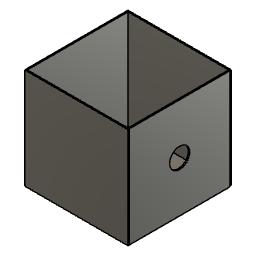
Rotating Flag Toy (Autodesk Fusion 360 archive; units mm, degrees)
design "gear1"
Autodesk Fusion 360 part; units mm, degrees
sketch "Sketch1" plane through (0, 0, 0) normal (0, 1, 0) x (1, 0, 0)
  line L0 (0, 0) -> (100, 0)
  line L1 (100, 0) -> (100, -100)
  line L2 (100, -100) -> (0, -100)
  line L3 (0, -100) -> (0, 0)
  constraint horizontal L0
  constraint vertical L1
  constraint horizontal L2
  constraint vertical L3
  constraint coincident L0.start L3.end
sketch "Sketch2" plane through (0, 0, 0) normal (0, 1, 0) x (1, 0, 0)
  line L0 (0, 0) -> (100, 0)
  line L1 (100, 0) -> (100, -100)
  line L2 (100, -100) -> (0, -100)
  line L3 (0, -100) -> (0, 0)
  constraint horizontal L0
  constraint vertical L1
  constraint horizontal L2
  constraint vertical L3
  constraint coincident L0.start L3.end
sketch "Sketch3" plane through (0, 0, 0) normal (0, 1, 0) x (1, 0, 0)
  line L0 (0, 0) -> (150, 0)
  line L1 (150, 0) -> (150, -150)
  line L2 (150, -150) -> (0, -150)
  line L3 (0, -150) -> (0, 0)
  dimension "d5" = 150
  dimension "d6" = 150
  constraint horizontal L0
  constraint vertical L1
  constraint horizontal L2
  constraint vertical L3
  constraint coincident L0.start L3.end
  measures "d5" distance of L0.start L0.end
  measures "d6" distance of L0.start L2.end
extrude "Extrude3" add sketch "Sketch3" along normal blind 2 makes body 1
sketch "Sketch4" plane through (150, 0, 0) normal (1, 0, 0) x (0, 0, -1)
  line L0 (-150, 0) -> (0, 0)
  line L1 (0, 0) -> (0, 2)
  line L2 (0, 2) -> (-150, 2)
  line L3 (-150, 2) -> (-150, 0)
  line L4 (0, 0) -> (-150, 0)
  line L5 (-150, 0) -> (-150, 150)
  line L6 (-150, 150) -> (0, 150)
  line L7 (0, 150) -> (0, 0)
  dimension "d9" = 150
  dimension "d10" = 150
  constraint horizontal L4
  constraint vertical L5
  constraint horizontal L6
  constraint vertical L7
  constraint coincident L0.end L1.start
  measures "d9" distance of L0.end L0.start
  measures "d10" distance of L0.end L6.end
extrude "Extrude4" add sketch "Sketch4" along normal blind 2 separate body contours L2 L5 L6 L7 makes body 2
move_face "OffsetFaces1" offset 2 1 faces at (151.3333, 2, 50) on bodies 2
sketch "Sketch5" plane through (0, 0, 0) normal (1, 0, 0) x (0, 0, -1)
  line L0 (0, 0) -> (-150, 0)
  line L1 (-150, 0) -> (-150, 150)
  line L2 (-150, 150) -> (0, 150)
  line L3 (0, 150) -> (0, 0)
  dimension "d14" = 150
  dimension "d15" = 150
  constraint horizontal L0
  constraint vertical L1
  constraint horizontal L2
  constraint vertical L3
  constraint coincident L0.start L3.end
  measures "d14" distance of L0.start L0.end
  measures "d15" distance of L0.start L2.end
extrude "Extrude5" add sketch "Sketch5" against normal blind 2 bodies 1
sketch "Sketch6" plane through (0, 0, 0) normal (0, 0, 1) x (1, 0, 0)
  line L0 (151.9625, 0.9965) -> (-1.993, 0.9965)
  line L1 (-1.993, 0.9965) -> (-1.993, 149.9695)
  line L2 (-1.993, 149.9695) -> (151.9625, 149.9695)
  line L3 (151.9625, 149.9695) -> (151.9625, 0.9965)
  constraint horizontal L0
  constraint vertical L1
  constraint horizontal L2
  constraint vertical L3
extrude "Extrude6" add sketch "Sketch6" against normal blind 2 bodies 1 2
ref_plane "WorkPlane1" through (0, 0, 150) normal (0, 0, 1) x (1, 0, 0)
sketch "Sketch7" plane through (0, 0, 150) normal (0, 0, 1) x (1, 0, 0)
  line L0 (0, 0) -> (151.9611, 0)
  line L1 (151.9611, 0) -> (151.9611, 149.9617)
  line L2 (151.9611, 149.9617) -> (0, 149.9617)
  line L3 (0, 149.9617) -> (0, 0)
  constraint horizontal L0
  constraint vertical L1
  constraint horizontal L2
  constraint vertical L3
  constraint coincident L0.start L3.end
extrude "Extrude7" add sketch "Sketch7" along normal blind 2 separate body makes body 3
move_face "OffsetFaces2" offset 2 1 faces at (0, 99.9744, 150.6667) on bodies 3
hole "Hole1" at (152, 75, 75) direction (-1, 0, 0) diameter 30 depth 50 tip angle 118 bodies 1

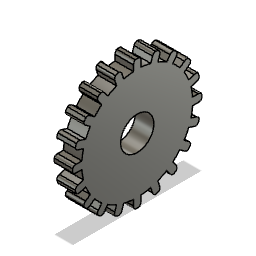
design "gear6"
Autodesk Fusion 360 part; units mm, degrees
sketch "Sketch1" plane through (0, 0, 0) normal (1, 0, 0) x (0, 0, -1)
  circle A0 centre (0, 0) radius 30
  dimension "d1" = 60
  constraint coincident A0.centre origin
  measures "d1" diameter of A0
extrude "Extrude1" add sketch "Sketch1" along normal blind 10
sketch "Sketch2" plane through (10, 0, 0) normal (1, 0, 0) x (0, 0, -1)
  circle A0 centre (0, 0) radius 30
  line L0 (-2.0249, 29.9316) -> (-2.0249, 33.0252)
  arc A1 (-1.0479, 34.9796) -> (-2.0249, 33.0252) centre (0.4183, 33.0252) ccw
  line L1 (-1.0479, 34.9796) -> (0.9463, 34.9796)
  arc A2 (2.0432, 33.0065) -> (0.9463, 34.9796) centre (0.0824, 33.2079) ccw
  line L2 (2.0432, 33.0065) -> (2.0432, 29.9303)
  constraint coincident A0 L0.start
  constraint vertical L0
  constraint tangent L0 A1
  constraint horizontal L1
  constraint coincident A0 L2.end
  constraint vertical L2
extrude "Extrude2" add sketch "Sketch2" against normal blind 10 contours A0 L0 A1 L1 A2 L2
pattern_circular "C-Pattern1" count 20 over 360 about axis through (0, 0, 0) along (1, 0, 0) of "Extrude2"
hole "Hole1" at (10, 0, 0) direction (-1, 0, 0) diameter 18 depth 18 tip angle 118

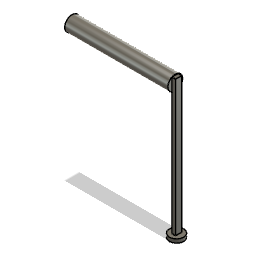
design "gear4"
Autodesk Fusion 360 part; units mm, degrees
sketch "Sketch1" plane through (0, 0, 0) normal (1, 0, 0) x (0, 0, -1)
  circle A0 centre (-15.9104, 20.2251) radius 10
  dimension "d1" = 20
  measures "d1" diameter of A0
extrude "Extrude1" add sketch "Sketch1" along normal blind 140
sketch "Sketch2" plane through (140, 0, 0) normal (1, 0, 0) x (0, 0, -1)
  circle A0 centre (-15.9104, 20.2251) radius 10
  line L0 (-20.4358, 29.1425) -> (-12.1034, 29.1425)
  line L1 (-12.1034, 29.1425) -> (-12.1034, -29.774)
  line L2 (-12.1034, -29.774) -> (-20.4358, -29.774)
  line L3 (-20.4358, -29.774) -> (-20.4358, 29.1425)
  constraint horizontal L0
  constraint vertical L1
  constraint horizontal L2
  constraint vertical L3
  constraint coincident A0 L0.start
extrude "Extrude2" add sketch "Sketch2" along normal blind 5 contours A0 L0 L1 L3 | A0 L1 L2 L3
extrude "Extrude3" add 1 faces at (141.6667, -29.774, 14.8809) along direction (0, -1, 0) blind 125
sketch "Sketch3" plane through (0, -154.774, 0) normal (0, -1, 0) x (1, 0, 0)
  line L0 (140, 20.4358) -> (140, 12.1034)
  line L1 (140, 12.1034) -> (145, 12.1034)
  line L2 (145, 12.1034) -> (145, 20.4358)
  line L3 (145, 20.4358) -> (140, 20.4358)
  circle A0 centre (142.5, 16.588) radius 9.71
extrude "Extrude4" add sketch "Sketch3" along normal blind 5 contours L0 L1 L2 L3 | A0

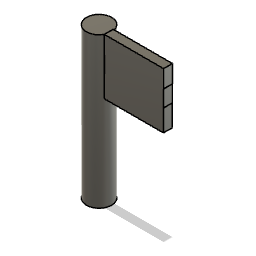
design "flag"
Autodesk Fusion 360 part; units mm, degrees
sketch "Sketch1" plane through (0, 0, 0) normal (0, 1, 0) x (1, 0, 0)
  circle A0 centre (0, 0) radius 4.263
  dimension "d1" = 8.526
  constraint coincident A0.centre origin
  measures "d1" diameter of A0
extrude "Extrude1" add sketch "Sketch1" along normal blind 51 makes body 1
sketch "Sketch2" plane through (0, 0, 0) normal (0, 0, 1) x (1, 0, 0)
  line L0 (4.2735, 51.0087) -> (19.9199, 51.0087)
  line L1 (19.9199, 51.0087) -> (19.9199, 45.0265)
  line L2 (19.9199, 45.0265) -> (4.2735, 45.0265)
  line L3 (4.2735, 45.0265) -> (4.2735, 51.0087)
  line L4 (4.2735, 45.0265) -> (19.9199, 45.0265)
  line L5 (19.9199, 45.0265) -> (19.9199, 39.038)
  line L6 (19.9199, 39.038) -> (4.2735, 39.038)
  line L7 (4.2735, 39.038) -> (4.2735, 45.0265)
  line L8 (4.2735, 39.038) -> (19.9199, 39.038)
  line L9 (19.9199, 39.038) -> (19.9199, 32.9058)
  line L10 (19.9199, 32.9058) -> (4.2735, 32.9058)
  line L11 (4.2735, 32.9058) -> (4.2735, 39.038)
  constraint horizontal L0
  constraint vertical L1
  constraint horizontal L2
  constraint vertical L3
  constraint horizontal L4
  constraint vertical L5
  constraint horizontal L6
  constraint vertical L7
  constraint horizontal L8
  constraint vertical L9
  constraint horizontal L10
  constraint vertical L11
extrude "Extrude2" add sketch "Sketch2" along normal blind 2 separate body contours L0 L1 L2 L3 L4 makes body 2
extrude "Extrude3" add 1 faces at (14.7044, 49.0146, 0) along direction (0, 0, -1) blind 1 on bodies 2 bodies 2
move_face "OffsetFaces1" offset 16 1 faces at (19.9199, 49.0146, 0) on bodies 2
move_face "OffsetFaces2" offset -12 1 faces at (35.9199, 49.0146, 0) on bodies 2
sketch "Sketch3" plane through (0, 0, 0) normal (0, 0, 1) x (1, 0, 0)
  line L0 (4.2852, 45.0296) -> (23.8847, 45.0296)
  line L1 (23.8847, 45.0296) -> (23.8847, 39.4097)
  line L2 (23.8847, 39.4097) -> (4.2852, 39.4097)
  line L3 (4.2852, 39.4097) -> (4.2852, 45.0296)
  constraint horizontal L0
  constraint vertical L1
  constraint horizontal L2
  constraint vertical L3
extrude "Extrude4" add sketch "Sketch3" along normal blind 2 bodies 2
move_face "OffsetFaces3" offset 1 1 faces at (10.8183, 43.1542, 0) on bodies 2
extrude "Extrude5" add 1 faces at (4.2852, 43.1542, 1) along direction (-1, 0, 0) blind 0.5 on bodies 2 bodies 2 1
extrude "Extrude6" add 1 faces at (4.2735, 47.0206, 0) along direction (-1, 0, 0) blind 0.5 on bodies 2 bodies 2
sketch "Sketch4" plane through (0, 0, 0) normal (0, 0, 1) x (1, 0, 0)
  line L0 (3.7832, 39.4209) -> (23.8708, 39.4209)
  line L1 (23.8708, 39.4209) -> (23.8708, 32.0868)
  line L2 (23.8708, 32.0868) -> (3.7832, 32.0868)
  line L3 (3.7832, 32.0868) -> (3.7832, 39.4209)
  constraint horizontal L0
  constraint vertical L1
  constraint horizontal L2
  constraint vertical L3
extrude "Extrude7" add sketch "Sketch4" along normal blind 2 bodies 2
extrude "Extrude8" add 1 faces at (10.7989, 34.5277, 0) along direction (0, 0, -1) blind 1 on bodies 2 bodies 2
